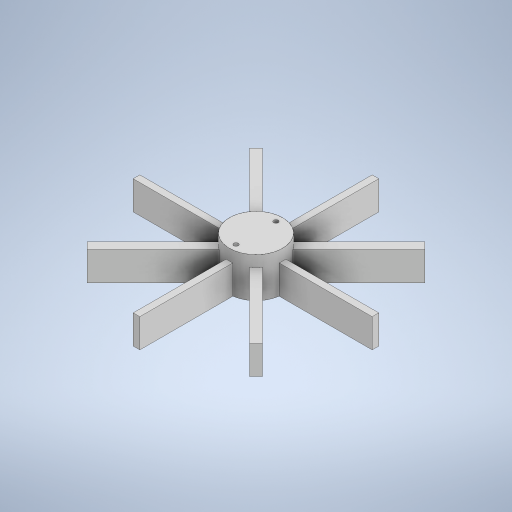
# Autodesk Inventor part: sweeper
Saved by Autodesk Inventor 2024 (Build 280153000, 153)
## iProperties
Created: 2024-05-20
Part Number: sweeper
Material: Generic
Document SubType Name: Modeling
Designer: ryana
Density: 1 g/cm^3
Appearance: Default
Author: ryana
Autodesk Inventor part; units mm, degrees
ref_plane "YZ Plane" through (0, 0, 0) normal (1, 0, 0) x (0, 1, 0)
ref_plane "XZ Plane" through (0, 0, 0) normal (0, 1, 0) x (-1, 0, 0)
ref_plane "XY Plane" through (0, 0, 0) normal (0, 0, 1) x (1, 0, 0)
sketch "Sketch2" plane through (0, 0, 0) normal (0, 1, 0) x (-1, 0, 0)
  circle A0 centre (0, 0) radius 12
  line L0 (-1.5, 54) -> (-1.5, -54)
  line L1 (-1.5, -54) -> (1.5, -54)
  line L2 (1.5, -54) -> (1.5, 54)
  line L3 (1.5, 54) -> (-1.5, 54)
  line L4 (-1.5, 54) -> (1.5, -54) construction
  line L5 (-1.5, -54) -> (1.5, 54) construction
  line L6 (-54, -1.5) -> (54, -1.5)
  line L7 (54, -1.5) -> (54, 1.5)
  line L8 (54, 1.5) -> (-54, 1.5)
  line L9 (-54, 1.5) -> (-54, -1.5)
  line L10 (-54, -1.5) -> (54, 1.5) construction
  line L11 (54, -1.5) -> (-54, 1.5) construction
  line L12 (1.5, 1.5) -> (-1.5, -1.5)
  line L13 (-1.5, -1.5) -> (36.6838, -39.6838)
  line L14 (36.6838, -39.6838) -> (39.6838, -36.6838)
  line L15 (39.6838, -36.6838) -> (1.5, 1.5)
  line L16 (1.5, 1.5) -> (-1.5, -1.5)
  line L17 (-1.5, -1.5) -> (-39.6838, 36.6838)
  line L18 (-39.6838, 36.6838) -> (-36.6838, 39.6838)
  line L19 (-36.6838, 39.6838) -> (1.5, 1.5)
  line L20 (-1.5, 1.5) -> (1.5, -1.5)
  line L21 (1.5, -1.5) -> (-36.6838, -39.6838)
  line L22 (-36.6838, -39.6838) -> (-39.6838, -36.6838)
  line L23 (-39.6838, -36.6838) -> (-1.5, 1.5)
  line L24 (-1.5, 1.5) -> (1.5, -1.5)
  line L25 (1.5, -1.5) -> (39.6838, 36.6838)
  line L26 (39.6838, 36.6838) -> (36.6838, 39.6838)
  line L27 (36.6838, 39.6838) -> (-1.5, 1.5)
  point P0 (6.8516, -9.8516)
  point P1 (9.8516, -6.8516)
  point P2 (11.9059, -1.5)
  point P3 (11.9059, 1.5)
  point P4 (9.8516, 6.8516)
  point P5 (6.8516, 9.8516)
  point P6 (1.5, 11.9059)
  point P7 (-1.5, 11.9059)
  point P8 (-6.8516, 9.8516)
  point P9 (-9.8516, 6.8516)
  point P10 (-11.9059, 1.5)
  point P11 (-11.9059, -1.5)
  point P12 (-9.8516, -6.8516)
  point P13 (-6.8516, -9.8516)
  point P14 (-1.5, -11.9059)
  point P15 (1.5, -11.9059)
  dimension "d0" = 24
  dimension "d1" = 108
  dimension "d2" = 3
  dimension "d3" = 108
  dimension "d4" = 3
  dimension "d5" = 54
  dimension "d6" = 54
  dimension "d7" = 54
  dimension "d8" = 54
  constraints: 56 end point, 12 parallel, 8 point on line, 6 perpendicular, 4 midpoint, 1 centre point, 1 coincident, 1 horizontal, 1 vertical
  measures "d0" diameter of A0
  measures "d1" distance of L0.start L0.end
  measures "d2" distance of L1.end L0.end
  measures "d3" distance of L6.start L6.end
  measures "d4" distance of L7.end L6.end
  measures "d5" distance of L13.end L12.end
  measures "d6" distance of L12.end L17.end
  measures "d7" distance of L20.end L21.end
  measures "d8" distance of L25.end L20.end
extrude "Extrusion1" add sketch "Sketch2" along normal blind 13
sketch "Sketch3" plane through (0, 13, 0) normal (0, 1, 0) x (1, 0, 0)
  arc A0 (-11.9059, -1.5) -> (-9.8516, -6.8516) centre (0, 0) ccw projected
  circle A1 centre (0, 0) radius 12
  point P0 (-9.8516, -6.8516)
  dimension "d11" = 24
  constraints: 1 centre point, 1 coincident
  measures "d11" diameter of A1
extrude "Extrusion2" add sketch "Sketch3" along normal blind 5
sketch "Sketch4" plane through (0, 18, 0) normal (0, 1, 0) x (1, 0, 0)
  line L0 (0, 0) -> (0, -12)
  circle A0 centre (0, 0) radius 12 projected
  line L1 (0, 0) -> (0, 12)
  line L2 (0, -12) -> (0, -9)
  line L3 (0, 12) -> (0, 9)
  circle A1 centre (0, -9) radius 1
  circle A2 centre (0, 9) radius 1
  dimension "d14" = 3
  dimension "d15" = 3
  dimension "d16" = 2
  dimension "d17" = 2
  constraints: 8 end point, 3 point on line, 2 centre point, 2 coincident, 2 point on circle, 1 vertical
  measures "d14" distance of L0.end L2.end
  measures "d15" distance of L1.end L3.end
  measures "d16" diameter of A1
  measures "d17" diameter of A2
extrude "Extrusion3" cut sketch "Sketch4" against normal blind 20 contours A1 L0 | L0 A1 | A2 L1 | L1 A2
body "Solid1"
